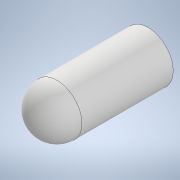
# Autodesk Inventor part: NotchPiston1
Saved by Autodesk Inventor 2021 (Build 250183000, 183)
## iProperties
Created: 2021-06-04
Part Number: NotchPiston1
Material: Generic
Document SubType Name: Modeling
Designer: teh18
Density: 1 g/cm^3
Appearance: Default
Author: teh18
Autodesk Inventor part; units mm, degrees
ref_plane "YZ Plane" through (0, 0, 0) normal (1, 0, 0) x (0, 1, 0)
ref_plane "XZ Plane" through (0, 0, 0) normal (0, 1, 0) x (-1, 0, 0)
ref_plane "XY Plane" through (0, 0, 0) normal (0, 0, 1) x (1, 0, 0)
sketch "Sketch1" plane through (0, 0, 0) normal (0, 0, 1) x (1, 0, 0)
  arc A0 (45.3033, 58.3033) -> (45.3033, 47.6967) centre (40, 53) ccw projected
  circle A1 centre (40, 53) radius 7.5
  circle A2 centre (40, 53) radius 7
  point P0 (0, 0)
  dimension "d3" = 0.5
  constraints: 2 centre point, 1 coincident, 1 concentric
  measures "d3" radial gap between concentric circles of A1 A2
extrude "Extrusion1" add sketch "Sketch1" along normal blind 40 contours A2
fillet "Fillet1" radius 7 1 edges at (33, 53, 40)
body "Solid1"
